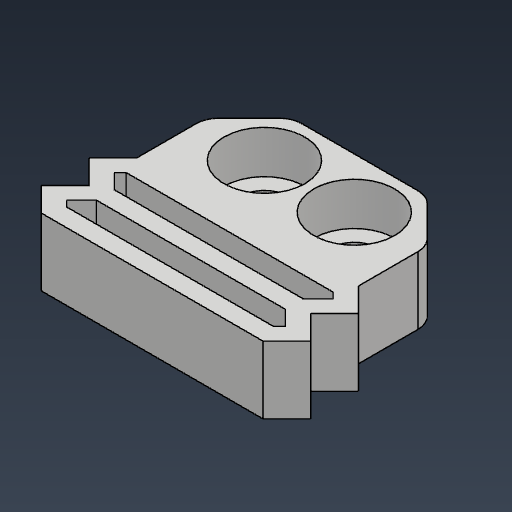
# Autodesk Inventor part: Kickerdaempfer
Saved by Autodesk Inventor 2023.1 (Build 271208000, 208)
## iProperties
Part Number: Kickerdaempfer
Material: Generisch
Document SubType Name: Modeling
Designer: rYan
Density: 1 g/cm^3
Appearance: Vorgabe
Mass: 1.43011 g
Surface Area: 17.3244 cm^2
Volume: 1.43011 cm^3
Author: rYan
Autodesk Inventor part; units mm, degrees
ref_plane "YZ Plane" through (0, 0, 0) normal (1, 0, 0) x (0, 1, 0)
ref_plane "XZ Plane" through (0, 0, 0) normal (0, 1, 0) x (-1, 0, 0)
ref_plane "XY Plane" through (0, 0, 0) normal (0, 0, 1) x (1, 0, 0)
sketch "Skizze3" plane through (0, 0, 0) normal (0, 0, 1) x (1, 0, 0)
  line L0 (0, 13.7) -> (0, -12.2) projected
  line L1 (-16.8, 0) -> (16.8, 0) projected
  circle A0 centre (4, 5.5) radius 2.1
  circle A1 centre (-4, 5.5) radius 2.1
  circle A2 centre (4, 5.5) radius 3.5 construction
  circle A3 centre (-4, 5.5) radius 3.5 construction
  line L2 (9.875, 0) -> (9.875, 6.125)
  line L3 (6, 10) -> (-6, 10)
  line L4 (-9.875, 6.125) -> (-9.875, 0)
  line L5 (9.875, 0) -> (-9.875, 0) construction
  line L6 (9.875, 0) -> (12, -2.125)
  line L7 (12, -2.125) -> (9.875, -4.25)
  line L8 (9.875, -4.25) -> (12, -6.375)
  line L9 (12, -6.375) -> (9.875, -8.5)
  line L10 (9.875, -8.5) -> (-9.875, -8.5)
  line L11 (-9.875, -8.5) -> (-12, -6.375)
  line L12 (-12, -6.375) -> (-9.875, -4.25)
  line L13 (-9.875, -4.25) -> (-12, -2.125)
  line L14 (-12, -2.125) -> (-9.875, 0)
  line L15 (12, -6.375) -> (-12, -6.375) construction
  line L16 (12, -2.125) -> (-12, -2.125) construction
  line L17 (9.875, 0) -> (9.875, -4.25) construction
  line L18 (12, -6.375) -> (12, -2.125) construction
  line L19 (9.7373, -6.375) -> (9.2123, -6.9)
  line L20 (9.2123, -6.9) -> (-9.2123, -6.9)
  line L21 (-9.2123, -6.9) -> (-9.7373, -6.375)
  line L22 (-9.7373, -6.375) -> (-8.4123, -5.05)
  line L23 (-8.4123, -5.05) -> (8.4123, -5.05)
  line L24 (8.4123, -5.05) -> (9.7373, -6.375)
  line L25 (9.7373, -2.125) -> (8.4123, -3.45)
  line L26 (8.4123, -3.45) -> (-8.4123, -3.45)
  line L27 (-8.4123, -3.45) -> (-9.7373, -2.125)
  line L28 (-9.7373, -2.125) -> (-9.2123, -1.6)
  line L29 (-9.2123, -1.6) -> (9.2123, -1.6)
  line L30 (9.2123, -1.6) -> (9.7373, -2.125)
  line L31 (9.875, -4.25) -> (-9.875, -4.25) construction
  line L32 (9.875, 6.125) -> (6, 10)
  line L33 (-9.875, 6.125) -> (-6, 10)
  point P0 (0, 0)
  dimension "d24" = 4.2
  dimension "d25" = 8
  dimension "d26" = 7
  dimension "d28" = 1
  dimension "d29" = 2
  dimension "d30" = 1.6
  dimension "d31" = 1.6
  dimension "d32" = 1.6
  dimension "d33" = 90
  dimension "d40" = 1.6
  dimension "d45" = 12
  dimension "d46" = 45
  dimension "d49" = 8.5
  dimension "d50" = 24
  constraints: 64 end point, 8 parallel, 5 horizontal, 5 point on line, 4 centre point, 3 vertical, 2 coincident, 2 perpendicular, 1 collinear, 20 other
  measures "d24" diameter of A0
  measures "d25" distance of A1.centre A0.centre
  measures "d26" diameter of A2
  measures "d28" distance edge to line of A2 L3
  measures "d29" distance edge to line of A2 L5
  measures "d30" distance between parallel lines of L10 L20
  measures "d31" distance between parallel lines of L9 L19
  measures "d32" distance between parallel lines of L7 L25
  measures "d33" angle of L19 L24
  measures "d40" distance between parallel lines of L26 L23
  measures "d45" distance of L3.start L3.end
  measures "d46" angle of L32 L3
  measures "d49" distance between parallel lines of L1 L10
  measures "d50" distance from line of L11.end L18
extrude "Extrusion2" add sketch "Skizze3" along normal blind 6 contours L3 L32 L2 L1 L0 | L0 L1 L4 L33 L3 | L1 L6 L7 L8 L9 L10 L0 L20 L19 L24 L23 L26 L25 L30 L29 | L0 L29 L28 L27 L26 L23 L22 L21 L20 L10 L11 L12 L13 L14 L1
sketch "Skizze4" plane through (0, 0, 6) normal (0, 0, 1) x (1, 0, 0)
  circle A0 centre (4, 5.5) radius 2.1 projected
  circle A1 centre (-4, 5.5) radius 2.1 projected
  circle A2 centre (4, 5.5) radius 3.6
  circle A3 centre (-4, 5.5) radius 3.6
  line L0 (0, 13.7) -> (0, -12.2) projected
  point P0 (0, 0)
  dimension "d37" = 7.2
  constraints: 2 centre point, 2 coincident, 1 other
  measures "d37" diameter of A2
extrude "Extrusion3" cut sketch "Skizze4" against normal blind 3.8
fillet "Rundung1" radius 2 4 edges at (9.875, 6.125, 3) (6, 10, 3) (-6, 10, 3) (-9.875, 6.125, 3)
equation "\"d31\" = d30"
equation "\"d32\" = d31"
equation "\"d40\" = d30"
